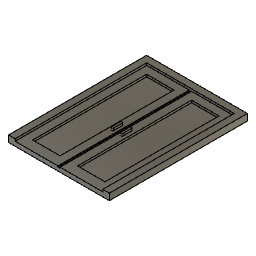
boardDoor (Autodesk Fusion 360 design; units mm, degrees)
Autodesk Fusion 360 part; units mm, degrees
sketch "Sketch1" plane through (0, 0, 0) normal (0, 0, 1) x (1, 0, 0)
  line L0 (131.7, 64.8) -> (131.7, 124.8)
  line L1 (91.7, 124.8) -> (91.7, 64.8)
  line L2 (131.7, 124.8) -> (91.7, 124.8)
  line L3 (91.7, 64.8) -> (131.7, 64.8)
  line L4 (131.7, 124.8) -> (91.7, 124.8)
  line L5 (131.7, 64.8) -> (131.7, 124.8)
  line L6 (91.7, 64.8) -> (131.7, 64.8)
  line L7 (91.7, 124.8) -> (91.7, 64.8)
  line L8 (131.7, 64.8) -> (131.7, 124.8)
  line L9 (91.7, 124.8) -> (91.7, 64.8)
  line L10 (131.7, 124.8) -> (91.7, 124.8)
  line L11 (91.7, 64.8) -> (131.7, 64.8)
  line L12 (131.7, 124.8) -> (91.7, 124.8)
  line L13 (131.7, 64.8) -> (131.7, 124.8)
  line L14 (91.7, 64.8) -> (131.7, 64.8)
  line L15 (91.7, 124.8) -> (91.7, 64.8)
  line L16 (131.7, 64.8) -> (131.7, 124.8)
  line L17 (91.7, 64.8) -> (131.7, 64.8)
  line L18 (91.7, 124.8) -> (91.7, 64.8)
  line L19 (131.7, 124.8) -> (91.7, 124.8)
  line L20 (131.7, 124.8) -> (91.7, 124.8)
  line L21 (131.7, 64.8) -> (131.7, 124.8)
  line L22 (131.7, 64.8) -> (131.7, 124.8)
  line L23 (91.7, 124.8) -> (91.7, 64.8)
  line L24 (91.7, 124.8) -> (91.7, 64.8)
  line L25 (131.7, 124.8) -> (91.7, 124.8)
  line L26 (91.7, 64.8) -> (131.7, 64.8)
  line L27 (131.7, 124.8) -> (91.7, 124.8)
  line L28 (91.7, 64.8) -> (131.7, 64.8)
  line L29 (131.7, 64.8) -> (131.7, 124.8)
  line L30 (91.7, 64.8) -> (131.7, 64.8)
  line L31 (91.7, 124.8) -> (91.7, 64.8)
  point P0 (129.8, 59.899)
  point P1 (93.6, 59.899)
  point P2 (129.8, 59.899)
  point P3 (93.6, 59.899)
sketch "Sketch2" plane through (0, 0, 0) normal (0, 0, 1) x (1, 0, 0)
  line L0 (131.7, 64.8) -> (131.7, 124.8)
  line L1 (88.7, 64.8) -> (134.7, 64.8)
  line L2 (88.7, 127.8) -> (88.7, 64.8)
  line L3 (134.7, 127.8) -> (88.7, 127.8)
  line L4 (131.7, 124.8) -> (110.7, 124.8)
  line L5 (131.7, 64.8) -> (131.7, 124.8)
  line L6 (134.7, 64.8) -> (134.7, 127.8)
  line L7 (131.7, 124.8) -> (112.7, 124.8)
  line L8 (112.7, 64.8) -> (131.7, 64.8)
  line L9 (131.7, 124.8) -> (91.7, 124.8)
  line L10 (110.7, 64.8) -> (131.7, 64.8)
  line L11 (131.7, 64.8) -> (131.7, 124.8)
  line L12 (91.7, 64.8) -> (131.7, 64.8)
  line L13 (91.7, 124.8) -> (91.7, 64.8)
sketch "Sketch6" plane through (0, 0, 0) normal (0, 0, 1) x (1, 0, 0)
  line L0 (111.2, 124.8) -> (111.2, 64.8)
  line L1 (112.2, 124.8) -> (112.2, 64.8)
  line L2 (111.2, 64.8) -> (112.2, 64.8)
  line L3 (111.2, 124.8) -> (112.2, 124.8)
  constraint perpendicular L1 L2
  constraint perpendicular L1 L3
sketch "Sketch7" plane through (0, 0, 0) normal (0, 0, 1) x (1, 0, 0)
  line L0 (95.2001, 121.3001) -> (107.7001, 121.3001)
  line L1 (107.7001, 121.3001) -> (107.7001, 69.3001)
  line L2 (107.7001, 69.3001) -> (95.2001, 69.3001)
  line L3 (95.2001, 69.3001) -> (95.2001, 121.3001)
  line L4 (95.2001, 121.3001) -> (107.7001, 121.3001)
  line L5 (107.7001, 121.3001) -> (107.7001, 69.3001)
  line L6 (95.2001, 69.3001) -> (95.2001, 121.3001)
  line L7 (115.7001, 121.3001) -> (128.2001, 121.3001)
  line L8 (128.2001, 121.3001) -> (128.2001, 69.3001)
  line L9 (115.7001, 69.3001) -> (115.7001, 121.3001)
  line L10 (128.2001, 69.3001) -> (115.7001, 69.3001)
  constraint horizontal L0
  constraint vertical L1
  constraint horizontal L2
  constraint vertical L3
  constraint horizontal L4
  constraint vertical L5
  constraint vertical L6
  constraint horizontal L7
  constraint vertical L8
  constraint horizontal L10
  constraint vertical L9
sketch "Sketch9" plane through (0, 0, 0) normal (0, 0, 1) x (1, 0, 0)
  line L0 (109.45, 96) -> (109.45, 96)
  line L1 (109.95, 95.5) -> (109.95, 91.5)
  line L2 (109.45, 91) -> (109.45, 91)
  line L3 (108.95, 91.5) -> (108.95, 95.5)
  line L4 (113.7, 96) -> (113.7, 96)
  line L5 (113.7, 91) -> (113.7, 91)
  line L6 (113.2, 91.5) -> (113.2, 95.5)
  line L7 (114.2, 95.5) -> (114.2, 91.5)
  arc A0 (109.45, 96) -> (108.95, 95.5) centre (109.45, 95.5) ccw
  arc A1 (109.95, 95.5) -> (109.45, 96) centre (109.45, 95.5) ccw
  arc A2 (113.7, 96) -> (113.2, 95.5) centre (113.7, 95.5) ccw
  arc A3 (114.2, 95.5) -> (113.7, 96) centre (113.7, 95.5) ccw
  arc A4 (113.7, 91) -> (114.2, 91.5) centre (113.7, 91.5) ccw
  arc A5 (113.2, 91.5) -> (113.7, 91) centre (113.7, 91.5) ccw
  arc A6 (109.45, 91) -> (109.95, 91.5) centre (109.45, 91.5) ccw
  arc A7 (108.95, 91.5) -> (109.45, 91) centre (109.45, 91.5) ccw
  dimension "d13" = 0.5
  constraint vertical L1
  constraint vertical L3
  constraint vertical L7
  constraint vertical L6
  constraint tangent L3 A0
  constraint tangent L1 A1
  constraint equal A0 A1
  constraint tangent L6 A2
  constraint equal A0 A2
  constraint tangent L7 A3
  constraint equal A0 A3
  constraint tangent L7 A4
  constraint equal A0 A4
  constraint tangent L6 A5
  constraint equal A0 A5
  constraint tangent L1 A6
  constraint equal A0 A6
  constraint tangent L3 A7
  constraint equal A0 A7
  measures "d13" radius of A0
extrude "Extrude1" add sketch "Sketch2" along normal blind 3 contours L0 L1 L2 L3 L4 L5 L6 L7 L9 L11 L13 makes body 1
extrude "Extrude2" add sketch "Sketch2" along normal blind 2 contours L0 L1 L4 L5 L7 L8 L9 L10 L11 L12 L13 bodies 1
form "Form1" [no effect]
extrude "Extrude3" add sketch "Sketch7" along normal blind 5 separate body contours L7 L8 L9 L10 makes body 2
extrude "Extrude4" add sketch "Sketch7" along normal blind 7 separate body contours L0 L1 L2 L3 L4 L5 L6 makes body 3
extrude "Extrude5" add sketch "Sketch6" along normal blind 11 separate body makes body 4
extrude "Extrude6" add sketch "Sketch9" along normal blind 13 separate body contours L1 L3 A0 A1 A6 A7 makes body 5
extrude "Extrude7" add sketch "Sketch9" along normal blind 13 separate body contours L6 L7 A2 A3 A4 A5 makes body 6
extrude "Extrude8" cut 1 faces at (124.0334, 86.6335, 5) along direction (0, 0, -1) blind 4 on bodies 2 bodies 1 2
extrude "Extrude9" cut 1 faces at (103.5334, 86.6335, 7) along direction (0, 0, -1) blind 6 on bodies 3 bodies 1 3
extrude "Extrude10" cut 1 faces at (111.5333, 104.8, 11) along direction (0, 0, -1) blind 9.5 on bodies 4 bodies 1 4
extrude "Extrude11" cut 1 faces at (113.5333, 94.1667, 13) along direction (0, 0, -1) blind 10 on bodies 6 bodies 6
extrude "Extrude12" cut 1 faces at (109.2833, 94.1667, 13) along direction (0, 0, -1) blind 10 on bodies 5 bodies 5
combine "Combine1" operation add target body 2 tool bodies 3 1 6 5 4
